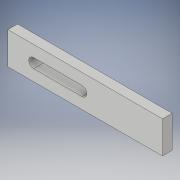
# Autodesk Inventor part: creat7
Saved by Autodesk Inventor 2019 (Build 230136000, 136)
## iProperties
Created: 2021-11-11
Part Number: creat7
Material: 一般
Document SubType Name: Modeling
Designer: yuta
Density: 1 g/cm^3
Appearance: 既定
Author: yuta
Autodesk Inventor part; units mm, degrees
ref_plane "YZ Plane" through (0, 0, 0) normal (1, 0, 0) x (0, 1, 0)
ref_plane "XZ Plane" through (0, 0, 0) normal (0, 1, 0) x (-1, 0, 0)
ref_plane "XY Plane" through (0, 0, 0) normal (0, 0, 1) x (1, 0, 0)
sketch "スケッチ1" plane through (0, 0, 0) normal (0, 0, 1) x (1, 0, 0)
  line L0 (-23.7126, 8.7959) -> (24.2874, 8.7959)
  line L1 (24.2874, 8.7959) -> (24.2874, -1.2041)
  line L2 (24.2874, -1.2041) -> (-23.7126, -1.2041)
  line L3 (-23.7126, -1.2041) -> (-23.7126, 8.7959)
  point P0 (0, 0)
  dimension "d0" = 48
  dimension "d1" = 10
  constraints: 8 end point, 2 parallel, 1 horizontal, 1 perpendicular
  measures "d0" distance of L1.end L2.end
  measures "d1" distance of L0.end L1.end
extrude "押し出し1" add sketch "スケッチ1" along normal blind 3
sketch "スケッチ2" plane through (0, 0, 3) normal (0, 0, 1) x (1, 0, 0)
  line L0 (-15.7126, 3.7959) -> (-0.7126, 3.7959) construction
  line L1 (-15.7126, 2.2959) -> (-0.7126, 2.2959)
  line L2 (-0.7126, 5.2959) -> (-15.7126, 5.2959)
  arc A0 (-15.7126, 5.2959) -> (-15.7126, 2.2959) centre (-15.7126, 3.7959) ccw
  arc A1 (-0.7126, 2.2959) -> (-0.7126, 5.2959) centre (-0.7126, 3.7959) ccw
  line L3 (-23.7126, 8.7959) -> (-23.7126, -1.2041) projected
  line L4 (24.2874, 8.7959) -> (-23.7126, 8.7959) projected
  point P0 (0, 0)
  point P1 (-8.2126, 3.7959)
  dimension "d4" = 15
  dimension "d5" = 3
  dimension "d6" = 8
  dimension "d7" = 5
  constraints: 8 end point, 4 point on circle, 4 tangent, 2 centre point, 1 horizontal, 1 midpoint, 1 parallel
  measures "d4" distance of L0.start L0.end
  measures "d5" diameter of A1
  measures "d6" distance from line of L3 L0.start
  measures "d7" distance from line of L4 L0.start
extrude "押し出し2" cut sketch "スケッチ2" against normal blind 3
